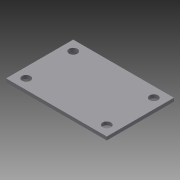
# Autodesk Inventor part: Caster_Plate
Saved by Autodesk Inventor 2014 (Build 180170000, 170)
## iProperties
Created: 2016-08-26
Part Number: Caster_Plate
Material: Generic
Document SubType Name: Modeling
Designer: jmw3
Density: 1 g/cm^3
Appearance: Default
Author: jmw3
Autodesk Inventor part; units mm, degrees
ref_plane "YZ Plane" through (0, 0, 0) normal (1, 0, 0) x (0, 1, 0)
ref_plane "XZ Plane" through (0, 0, 0) normal (0, 1, 0) x (-1, 0, 0)
ref_plane "XY Plane" through (0, 0, 0) normal (0, 0, 1) x (1, 0, 0)
sketch "Sketch1" plane through (0, 0, 0) normal (0, 1, 0) x (-1, 0, 0)
  line L0 (0, -44.45) -> (0, 44.45) projected
  line L1 (66.675, 0) -> (-66.675, 0) projected
  line L2 (47.625, -31.75) -> (-47.625, -31.75)
  line L3 (-47.625, -31.75) -> (-47.625, 31.75)
  line L4 (-47.625, 31.75) -> (47.625, 31.75)
  line L5 (47.625, 31.75) -> (47.625, -31.75)
  circle A0 centre (38.1, -22.225) radius 3.9688
  circle A1 centre (38.1, 22.225) radius 3.9688
  circle A2 centre (-38.1, -22.225) radius 3.9688
  circle A3 centre (-38.1, 22.225) radius 3.9688
  point P0 (0, 0)
  dimension "d0" = 95.25
  dimension "d1" = 63.5
  dimension "d2" = 38.1
  dimension "d3" = 22.225
  dimension "d4" = 7.9375
  constraints: 8 end point, 4 centre point, 3 symmetric about line, 2 parallel, 1 horizontal, 1 perpendicular, 5 other
  measures "d0" distance of L3.end L4.end
  measures "d1" distance between parallel lines of L4 L2
  measures "d2" distance from line of L0 A0.centre
  measures "d3" distance from line of L1 A0.centre
  measures "d4" diameter of A0
extrude "Extrusion1" add sketch "Sketch1" along normal blind 3.175
body "Solid1"
